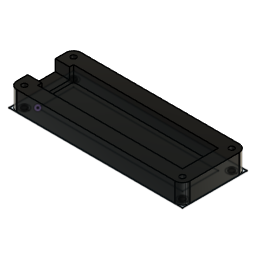
copypasy v2 (Autodesk Fusion 360 design; units mm, degrees)
Autodesk Fusion 360 part; units mm, degrees
sketch "Sketch1" plane through (0, 0, 0) normal (0, 0, 1) x (1, 0, 0) in component "WeCopy"
  line L0 (0, 0) -> (96.62, 0)
  line L1 (96.62, 0) -> (96.62, 23.86)
  line L2 (96.62, 23.86) -> (0, 23.86)
  line L3 (0, 23.86) -> (0, 0)
  line L4 (-9.5, -9.5) -> (106.12, -9.5)
  line L5 (106.12, -9.5) -> (106.12, 33.36)
  line L6 (106.12, 33.36) -> (-9.5, 33.36)
  line L7 (-9.5, 33.36) -> (-9.5, -9.5)
  circle A0 centre (101.12, 28.36) radius 1.7
  circle A1 centre (101.12, -4.5) radius 1.7
  circle A2 centre (-4.5, 28.36) radius 1.7
  circle A3 centre (-4.5, -4.5) radius 1.7
  circle A4 centre (101.12, 28.36) radius 3
  circle A5 centre (101.12, -4.5) radius 3
  circle A6 centre (-4.5, -4.5) radius 3
  circle A7 centre (-4.5, 28.36) radius 3
  dimension "d1" = 96.62
  dimension "d2" = 23.86
  dimension "d3" = 115.62
  dimension "d4" = 42.86
  dimension "d5" = 9.5
  dimension "d6" = 9.5
  dimension "d7" = 9.5
  dimension "d8" = 9.5
  dimension "d9" = 3.4
  dimension "d10" = 3.4
  dimension "d11" = 3.4
  dimension "d12" = 3.4
  dimension "d13" = 5
  dimension "d14" = 5
  dimension "d15" = 5
  dimension "d16" = 5
  dimension "d17" = 5
  dimension "d18" = 5
  dimension "d19" = 5
  dimension "d20" = 5
  dimension "d21" = 6
  dimension "d22" = 6
  dimension "d23" = 6
  dimension "d24" = 6
  constraint horizontal L0
  constraint vertical L1
  constraint horizontal L2
  constraint vertical L3
  constraint coincident L0.start L3.end
  constraint horizontal L4
  constraint vertical L5
  constraint horizontal L6
  constraint vertical L7
  constraint concentric A0 A4
  constraint concentric A1 A5
  constraint concentric A3 A6
  constraint concentric A2 A7
  measures "d1" distance of L0.start L0.end
  measures "d2" distance of L0.start L2.end
  measures "d3" distance of L4.start L4.end
  measures "d4" distance of L4.start L6.end
  measures "d5" distance of L2 L6
  measures "d6" distance of L1 L5
  measures "d7" distance of L0 L4
  measures "d8" distance of L3 L7
  measures "d9" diameter of A0
  measures "d10" diameter of A1
  measures "d11" diameter of A2
  measures "d12" diameter of A3
  measures "d13" distance of L6 A2.centre
  measures "d14" distance of L7 A2.centre
  measures "d15" distance of L4 A3.centre
  measures "d16" distance of L7 A3.centre
  measures "d17" distance of L4 A1.centre
  measures "d18" distance of L5 A1.centre
  measures "d19" distance of L6 A0.centre
  measures "d20" distance of L5 A0.centre
  measures "d21" diameter of A4
  measures "d22" diameter of A5
  measures "d23" diameter of A6
  measures "d24" diameter of A7
extrude "Extrude2" add sketch "Sketch1" along normal blind 9.9 from surface at 3.1 contours A4 | A5 | A6 | A7 makes body 1 at (99.7514, 25.6904, 6.4) makes body 2 at (-1.5037, -4.6495, 9.7) makes body 3 at (101.9325, -1.6121, 9.7) makes body 4 at (-1.5037, 28.2105, 9.7) in component "WeCopy"
extrude "Extrude3" add sketch "Sketch1" along normal blind 13 contours L4 L5 L6 L7 bodies 1 2 3 4 in component "WeCopy"
extrude "Extrude4" add sketch "Sketch1" along normal blind 3 contours L0 L1 L2 L3 bodies 1 in component "WeCopy"
sketch "Sketch2" plane through (0, 0, 3) normal (0, 0, 1) x (-1, 0, 0) in component "WeCopy"
  line L0 (0, -23.86) -> (0, 0)
  line L1 (0, 0) -> (-96.62, 0)
  line L2 (-96.62, 0) -> (-96.62, -23.86)
  line L3 (-96.62, -23.86) -> (0, -23.86)
  line L4 (14, -21.2325) -> (-4.5, -21.2325)
  line L5 (-4.5, -21.2325) -> (-4.5, -2.7325)
  line L6 (-4.5, -2.7325) -> (14, -2.7325)
  line L7 (14, -2.7325) -> (14, -21.2325)
  line L8 (9.5, 9.5) -> (-106.12, 9.5)
  dimension "d35" = 18.5
  dimension "d36" = 18.5
  dimension "d37" = 12.2325
  constraint horizontal L4
  constraint vertical L5
  constraint horizontal L6
  constraint vertical L7
  measures "d35" distance of L4.start L4.end
  measures "d36" distance of L4.start L6.end
  measures "d37" distance of L6 L8
extrude "Extrude5" cut sketch "Sketch2" against normal blind 7.5 from surface at 10 contours L0 L4 L6 L7 bodies 1 in component "WeCopy"
fillet "Fillet1" radius 5 1 edges at (-9.5, 33.36, 6.5) on bodies 1 in component "WeCopy"
fillet "Fillet2" radius 5 1 edges at (-9.5, -9.5, 6.5) on bodies 1 in component "WeCopy"
fillet "Fillet3" radius 5 1 edges at (106.12, -9.5, 6.5) on bodies 1 in component "WeCopy"
fillet "Fillet4" radius 5 1 edges at (106.12, 33.36, 6.5) on bodies 1 in component "WeCopy"
component "WeCopy" placed x (1, 0, 0) y (0, 1, 0) z (0, 0, 1) at (0, 0, 0)
